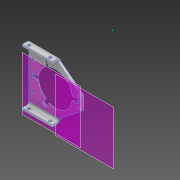
# Autodesk Inventor part: bearingcover
Saved by Autodesk Inventor 2018 (Build 220112000, 112)
## iProperties
Created: 2018-06-15
Part Number: bearingcover
Material: アルミニウム 6061
Document SubType Name: Sheet Metal
Designer: NaMACHAN
Density: 2.7 g/cm^3
Sheet Metal Rule: Default
Appearance: アルミニウム - フラット
Mass: 7.40744 g
Surface Area: 36.6566 cm^2
Volume: 2.7435 cm^3
Flat Pattern Width: 5 cm
Flat Pattern Length: 6.30478 cm
Flat Pattern Area: 31.5239 cm^2
Sheet Metal Width: 50.000 mm
Sheet Metal Length: 63.048 mm
Sheet Metal Area: 3152.389 mm^2
Author: NaMACHAN
Autodesk Inventor part; units mm, degrees
ref_plane "YZ Plane" through (0, 0, 0) normal (1, 0, 0) x (0, 1, 0)
ref_plane "XZ Plane" through (0, 0, 0) normal (0, 1, 0) x (-1, 0, 0)
ref_plane "XY Plane" through (0, 0, 0) normal (0, 0, 1) x (1, 0, 0)
ref_plane "作業平面1" through (-13.0598, -47.8022, -11.0593) normal (0, 1, 0) x (-1, 0, 0)
ref_plane "作業平面2" through (18.0823, -47.8022, -13) normal (0, 1, 0) x (-1, 0, 0)
sketch "スケッチ15" plane through (18.0823, -47.8022, -13) normal (0, 1, 0) x (-1, 0, 0)
  arc A0 (34.2516, 0.2523) -> (40.4568, 11) centre (24.5823, 13) ccw
  arc A1 (8.7078, 11) -> (30.7875, -1.7477) centre (24.5823, 13) ccw
  arc A2 (30.7875, 27.7477) -> (8.7078, 15) centre (24.5823, 13) ccw
  arc A3 (40.4568, 15) -> (34.2516, 25.7477) centre (24.5823, 13) ccw
  line L0 (46.5823, 11) -> (44.0823, 11)
  line L1 (44.0823, 15) -> (46.5823, 15)
  line L2 (37.0643, 30.6195) -> (36.0643, 28.8875)
  line L3 (32.6002, 30.8875) -> (33.6002, 32.6195)
  line L4 (3.0823, 15) -> (5.0823, 15)
  line L5 (5.0823, 11) -> (3.0823, 11)
  line L6 (3.0823, 11) -> (3.0823, 15)
  line L7 (46.5823, 15) -> (46.5823, 11)
  line L8 (33.6002, 32.6195) -> (37.0643, 30.6195)
  line L9 (37.3143, -5.0526) -> (33.8502, -7.0526)
  line L10 (33.8502, -7.0526) -> (32.6002, -4.8875)
  line L11 (36.0643, -2.8875) -> (37.3143, -5.0526)
  circle A4 centre (45.5823, 26) radius 1.5
  circle A5 centre (45.5823, 0) radius 1.5
  line L12 (21.5823, 36) -> (-0.4177, 19)
  line L13 (-0.4177, 19) -> (-0.4177, 7)
  line L14 (-0.4177, 7) -> (21.5823, -10)
  line L15 (49.5823, -4) -> (49.5823, 30)
  circle A6 centre (2.5823, 18) radius 1.5
  circle A7 centre (2.5823, 8) radius 1.5
  line L16 (5.0823, 11) -> (8.7078, 11)
  line L17 (5.0823, 15) -> (8.7078, 15)
  line L18 (36.0643, -2.8875) -> (34.2516, 0.2523)
  line L19 (30.7875, -1.7477) -> (32.6002, -4.8875)
  line L20 (40.4568, 11) -> (44.0823, 11)
  line L21 (44.0823, 15) -> (40.4568, 15)
  line L22 (34.2516, 25.7477) -> (36.0643, 28.8875)
  line L23 (32.6002, 30.8875) -> (30.7875, 27.7477)
  line L24 (49.5823, -4) -> (49.5823, -14)
  line L25 (49.5823, -14) -> (21.5823, -14)
  line L26 (21.5823, -14) -> (21.5823, -10)
  line L27 (21.5823, 36) -> (21.5823, 40)
  line L28 (21.5823, 40) -> (49.5823, 40)
  line L29 (49.5823, 40) -> (49.5823, 30)
  point P0 (18.0823, 13)
  dimension "d79" = 10
  dimension "d80" = 10
  measures "d79" distance of L15.start L24.end
  measures "d80" distance of L28.end L15.end
extrude "プレート6" add sketch "スケッチ15" along normal blind 2
chamfer "面取り4" distance 2 angle 45 4 edges at (-20.3564, -45.8022, -8) (-20.3564, -45.8022, 8) (1.5, -45.8022, 13.8564) (1.5, -45.8022, -13.8564)
sketch "スケッチ16" plane through (-31.5, -47.8022, 27) normal (0, 0, 1) x (1, 0, 0)
  point P0 (31.5, 47.8022)
sketch "スケッチ17" plane through (-31.5, -45.8022, 25) normal (0, 0, 1) x (1, 0, 0)
  line L0 (28, 0) -> (0, 0)
  line L1 (0, 0) -> (0, -8)
  line L2 (0, -8) -> (28, -8)
  line L3 (28, -8) -> (28, 0)
  constraints: 6 end point, 1 horizontal, 1 perpendicular, 1 vertical
edge flange "フランジ2" height 8 angle 90 thickness 2 bend radius 2 thickness toward (0, 0, 1) relief straight relief width 2 relief depth 1 corner gap 2 corner form 0 edges at (-17.5, -47.8022, 27) (-17.5, -47.8022, -27) wall of the first edge with corners at (-3.5, -45.8022, 25) (-31.5, -45.8022, 25) (-31.5, -53.8022, 25) (-3.5, -53.8022, 25)
bend "曲げ2"
corner "コーナー2"
sketch "スケッチ18" plane through (-31.5, -53.8022, 27) normal (0, 0, 1) x (1, 0, 0)
  line L0 (28, 4) -> (28, 0) projected
  line L1 (0, 0) -> (0, 4) projected
  point P0 (31.5, 53.8022)
  point P1 (24, 2)
  point P2 (4, 2)
  point P3 (28, 2)
  point P4 (0, 2)
  dimension "d95" = 4
  dimension "d96" = 4
  constraints: 3 horizontal alignment, 2 midpoint
  measures "d95" distance from line of L0 point (24, 2)
  measures "d96" distance from line of L1 point (4, 2)
hole "穴4" at (-27.5, -51.8022, 27) at (-7.5, -51.8022, 27) direction (0, 0, -1) diameter 3 end through all
equation "\"d102\" = Thickness"
equation "\"d81\" = Thickness"
equation "\"d85\" = BendReliefWidth"
equation "\"d86\" = BendReliefDepth"
equation "\"d87\" = MinimumRemnant"
equation "\"d88\" = TransitionRadius"
equation "\"d91\" = BendRadius"
equation "\"d92\" = CornerReliefSize"
equation "\"d93\" = GapSize"
equation "\"d94\" = JacobiRadiusSize"
equation "\"BendRadius\" = Thickness"
equation "\"BendReliefWidth\" = Thickness"
equation "\"BendReliefDepth\" = 0.5 * Thickness"
equation "\"CornerReliefSize\" = 4 * Thickness"
equation "\"MinimumRemnant\" = 2 * Thickness"
equation "\"TransitionRadius\" = BendRadius"
equation "\"JacobiRadiusSize\" = Thickness"
equation "\"GapSize\" = Thickness"
equation "\"Thickness\" = 2"
